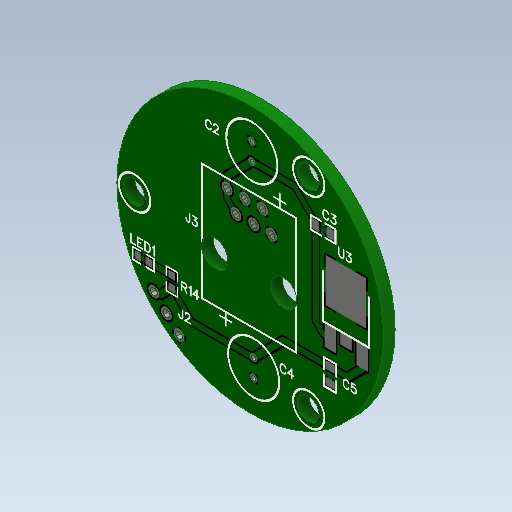
# Autodesk Inventor part: Power Supply
Saved by Autodesk Inventor 2020 (Build 240168000, 168)
## iProperties
Created: 2018-03-28
Part Number: Power Supply
Material: Generic
Document SubType Name: Modeling
Designer: Alex
Density: 1 g/cm^3
Appearance: Default
Mass: 1.79129 g
Surface Area: 25.1709 cm^2
Volume: 1.79129 cm^3
Author: Alex
Autodesk Inventor part; units mm, degrees
ref_plane "YZ Plane" through (0, 0, 0) normal (1, 0, 0) x (0, 1, 0)
ref_plane "XZ Plane" through (0, 0, 0) normal (0, 1, 0) x (-1, 0, 0)
ref_plane "XY Plane" through (0, 0, 0) normal (0, 0, 1) x (1, 0, 0)
sketch "Sketch1" plane through (0, 0, 0) normal (0, 0, 1) x (1, 0, 0)
  circle A0 centre (0, 0) radius 19.05
  dimension "d0" = 38.1
  constraints: 1 centre point, 1 coincident
  measures "d0" diameter of A0
extrude "Extrusion1" add sketch "Sketch1" along normal blind 1.651
sketch "Sketch2" plane through (0, 0, 1.651) normal (0, 0, 1) x (1, 0, 0)
  circle A0 centre (0, 0) radius 19.05 projected
  line L0 (-19.05, 19.05) -> (19.05, 19.05) construction
  line L1 (19.05, 19.05) -> (19.05, -19.05) construction
  line L2 (19.05, -19.05) -> (-19.05, -19.05) construction
  line L3 (-19.05, -19.05) -> (-19.05, 19.05) construction
  point P0 (-19.05, 0)
  point P1 (0, 19.05)
  constraints: 2 midpoint, 1 horizontal, 1 horizontal alignment, 1 tangent, 1 vertical alignment, 2 other
decal "Decal1"
sketch "Sketch3" plane through (0, 0, 0) normal (0, 0, -1) x (-1, 0, 0)
  circle A0 centre (0, 0) radius 19.05 projected
  line L0 (-19.05, 19.05) -> (19.05, 19.05) construction
  line L1 (19.05, 19.05) -> (19.05, -19.05) construction
  line L2 (19.05, -19.05) -> (-19.05, -19.05) construction
  line L3 (-19.05, -19.05) -> (-19.05, 19.05) construction
  point P0 (-19.05, 0)
  point P1 (0, 19.05)
  constraints: 2 midpoint, 1 horizontal, 1 horizontal alignment, 1 tangent, 1 vertical alignment, 2 other
decal "Decal2"
sketch "Sketch4" plane through (0, 0, 1.651) normal (0, 0, 1) x (1, 0, 0)
  circle A0 centre (-16.5947, 0) radius 1.5875
  circle A1 centre (8.2973, -14.3714) radius 1.5875
  circle A2 centre (8.2973, 14.3714) radius 1.5875
  line L0 (-16.5947, 0) -> (8.2973, 14.3714) construction
  line L1 (8.2973, 14.3714) -> (8.2973, -14.3714) construction
  line L2 (8.2973, -14.3714) -> (-16.5947, 0) construction
  line L3 (19.05, -19.05) -> (-19.05, -19.05) construction
  line L4 (-19.05, -19.05) -> (-19.05, 19.05) construction
  line L5 (-19.05, 19.05) -> (19.05, 19.05) construction
  line L6 (19.05, 19.05) -> (19.05, -19.05) construction
  line L7 (19.05, -19.05) -> (-19.05, 19.05) construction
  line L8 (-19.05, -19.05) -> (19.05, 19.05) construction
  circle A3 centre (0, 0) radius 19.05 construction
  circle A4 centre (0, 0) radius 19.05 construction
  circle A5 centre (-3.302, 7.112) radius 0.508
  circle A6 centre (-0.762, 7.112) radius 0.508
  circle A7 centre (1.778, 7.112) radius 0.508
  circle A8 centre (3.048, 4.572) radius 0.508
  circle A9 centre (0.508, 4.572) radius 0.508
  circle A10 centre (-2.032, 4.572) radius 0.508
  circle A11 centre (0.2794, 12.2174) radius 0.3175
  circle A12 centre (0.2794, 14.732) radius 0.3175
  circle A13 centre (-13.7521, -10.8859) radius 0.508
  circle A14 centre (-11.9561, -12.6819) radius 0.508
  circle A15 centre (-10.16, -14.478) radius 0.508
  line L9 (-13.7521, -10.8859) -> (-10.16, -14.478) construction
  line L10 (-10.16, -14.478) -> (-15.24, -14.478) construction
  circle A16 centre (0.508, -11.9634) radius 0.3175
  circle A17 centre (0.508, -14.478) radius 0.3175
  circle A18 centre (-5.08, -1.778) radius 1.905
  circle A19 centre (4.7752, -1.778) radius 1.905
  point P0 (0, 19.05)
  point P1 (-19.05, 0)
  dimension "d8" = 3.175
  dimension "d9" = 2.54
  dimension "d10" = 2.54
  dimension "d11" = 2.54
  dimension "d12" = 1.27
  dimension "d13" = 2.54
  dimension "d14" = 2.54
  dimension "d15" = 1.016
  dimension "d16" = 11.938
  dimension "d17" = 15.748
  dimension "d18" = 0.635
  dimension "d19" = 0.635
  dimension "d20" = 4.318
  dimension "d21" = 2.5146
  dimension "d22" = 19.3294
  dimension "d23" = 1.016
  dimension "d26" = 5.08
  dimension "d27" = 45
  dimension "d28" = 4.572
  dimension "d29" = 8.89
  dimension "d30" = 0.635
  dimension "d31" = 0.635
  dimension "d32" = 2.5146
  dimension "d33" = 4.572
  dimension "d34" = 19.558
  dimension "d35" = 9.8552
  dimension "d36" = 3.81
  dimension "d37" = 13.97
  dimension "d38" = 20.828
  dimension "d41" = 24.892
  dimension "d42" = 4.6786
  dimension "d43" = 33.4214
  dimension "d44" = 27.3473
  constraints: 22 end point, 18 centre point, 10 equal radius, 7 horizontal alignment, 5 coincident, 5 midpoint, 3 vertical alignment, 2 horizontal, 2 parallel, 1 equal length, 1 perpendicular, 9 other
  measures "d8" diameter of A0
  measures "d9" distance of A6.centre A5.centre
  measures "d10" distance of A7.centre A6.centre
  measures "d11" vertical distance of A10.centre A5.centre
  measures "d12" horizontal distance of A10.centre A5.centre
  measures "d13" distance of A9.centre A10.centre
  measures "d14" distance of A8.centre A9.centre
  measures "d15" diameter of A5
  measures "d16" distance from line of L5 A5.centre
  measures "d17" distance from line of L4 A5.centre
  measures "d18" diameter of A11
  measures "d19" diameter of A12
  measures "d20" distance from line of L5 A12.centre
  measures "d21" distance of A12.centre A11.centre
  measures "d22" distance from line of L4 A12.centre
  measures "d23" diameter of A14
  measures "d26" distance of L9.end L10.end
  measures "d27" angle of L10 L9
  measures "d28" distance between parallel lines of L3 L10
  measures "d29" distance from line of L4 L9.end
  measures "d30" diameter of A16
  measures "d31" diameter of A17
  measures "d32" distance of A17.centre A16.centre
  measures "d33" distance from line of A17.centre L3
  measures "d34" distance from line of L4 A17.centre
  measures "d35" distance of A19.centre A18.centre
  measures "d36" diameter of A18
  measures "d37" distance from line of L4 A18.centre
  measures "d38" distance from line of L5 A18.centre
  measures "d41" distance from line of A0.centre L1
  measures "d42" distance from line of L5 A2.centre
  measures "d43" distance from line of L5 A1.centre
  measures "d44" distance from line of L4 L0.end
extrude "Extrusion2" cut sketch "Sketch4" against normal through all
equation "\"d30\" = d31"
body "Solid1"
